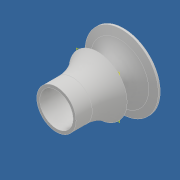
# Autodesk Inventor part: soundcone
Saved by Autodesk Inventor 2017 (Build 210142000, 142)
## iProperties
Created: 2017-09-21
Part Number: soundcone
Material: Generic
Document SubType Name: Modeling
Designer: Josh
Density: 1 g/cm^3
Appearance: Default
Author: Josh
Autodesk Inventor part; units mm, degrees
ref_plane "YZ Plane" through (0, 0, 0) normal (1, 0, 0) x (0, 1, 0)
ref_plane "XZ Plane" through (0, 0, 0) normal (0, 1, 0) x (-1, 0, 0)
ref_plane "XY Plane" through (0, 0, 0) normal (0, 0, 1) x (1, 0, 0)
sketch "Sketch1" plane through (0, 0, 0) normal (1, 0, 0) x (0, 1, 0)
  line L0 (0, -8.5) -> (13, -8.5)
  line L1 (21.2076, -14.7796) -> (32.2076, -14.7796)
  line L2 (16, 0) -> (0, 0)
  line L3 (0, 0) -> (0, -8.5)
  arc A0 (32.2076, -14.7796) -> (16, 0) centre (12.8346, -19.7479) ccw
  arc A1 (21.2076, -14.7796) -> (13, -8.5) centre (13, -17.0036) ccw
  line L4 (8.2331, -10) -> (0, -10)
  arc A2 (21.2076, -14.7796) -> (8.2331, -10) centre (8.2331, -30) ccw
  line L5 (0, -8.5) -> (0, -10)
  line L6 (32.2076, -14.7796) -> (33.2013, -18.6542)
  line L7 (33.2013, -18.6542) -> (34.2013, -18.6542)
  line L8 (16, 0) -> (29, 0)
  arc A3 (34.2013, -18.6542) -> (29, 0) centre (-1.8506, -18.6542) ccw
  dimension "d2" = 16
  dimension "d3" = 8.5
  dimension "d4" = 13
  dimension "d7" = 20
  dimension "d8" = 11
  dimension "d9" = 1.5
  dimension "d71" = 1
  dimension "d72" = 4
  dimension "d73" = 20
  dimension "d74" = 13
  constraints: 18 end point, 8 point on circle, 4 centre point, 4 horizontal, 3 tangent, 1 line through centre, 1 parallel, 1 perpendicular, 1 vertical, 1 other
  measures "d2" distance of L2.start L2.end
  measures "d3" distance of L2.end L0.start
  measures "d4" distance of L0.start L0.end
  measures "d7" distance of L1.end A0.centre
  measures "d8" distance of L1.start L1.end
  measures "d9" distance between parallel lines of L0 L4
  measures "d71" distance of L6.end L7.end
  measures "d72" distance of L1.end L6.end
  measures "d73" radius of A2
  measures "d74" distance of L2.start L8.end
revolve "Revolution3" add sketch "Sketch1" angle 360 about axis through (0, 16, 0) along (0, -1, 0) contours L0 A1 A2 L4 L5 | L8 A3 L7 L6 A0
ref_plane "Work Plane2" through (0, 21.25, 0) normal (0, -1, 0) x (1, 0, 0)
body "Solid2"
